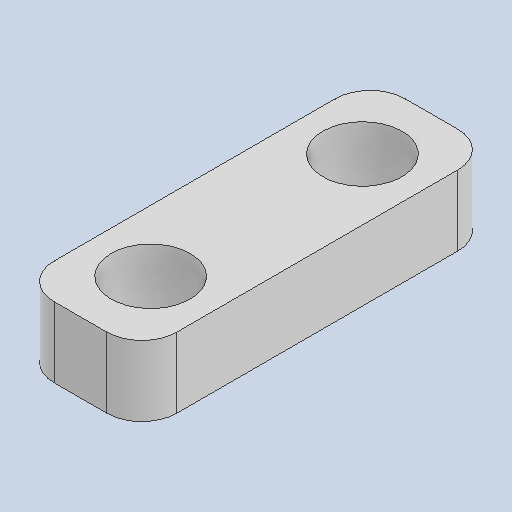
# Autodesk Inventor part: Aparter
Saved by Autodesk Inventor 2025 (Build 290162000, 162)
## iProperties
Created: 2025-08-11
Part Number: Aparter
Material: Generic
Document SubType Name: Modeling
Designer: Pravoslav
Density: 1 g/cm^3
Appearance: Default
Author: Pravoslav
Autodesk Inventor part; units mm, degrees
ref_plane "YZ Plane" through (0, 0, 0) normal (1, 0, 0) x (0, 1, 0)
ref_plane "XZ Plane" through (0, 0, 0) normal (0, 1, 0) x (-1, 0, 0)
ref_plane "XY Plane" through (0, 0, 0) normal (0, 0, 1) x (1, 0, 0)
sketch "Sketch1" plane through (0, 0, 0) normal (0, 1, 0) x (-1, 0, 0)
  circle A0 centre (-0.5725, 7.3819) radius 2.25
  circle A1 centre (-0.5725, -4.6791) radius 2.25
  line L0 (2.9275, 11.3819) -> (-4.0725, 11.3819)
  line L1 (-4.0725, 11.3819) -> (-4.0725, -8.6181)
  line L2 (-4.0725, -8.6181) -> (2.9275, -8.6181)
  line L3 (2.9275, -8.6181) -> (2.9275, 11.3819)
  point P0 (0, 0)
  dimension "d0" = 4.5
  dimension "d1" = 4.5
  dimension "d2" = 12.061
  dimension "d3" = 7
  dimension "d4" = 3.5
  dimension "d5" = 20
  dimension "d6" = 4
  constraints: 8 end point, 2 centre point, 2 parallel, 1 horizontal, 1 perpendicular
  measures "d0" diameter of A0
  measures "d1" diameter of A1
  measures "d2" distance of A1.centre A0.centre
  measures "d3" distance between parallel lines of L1 L3
  measures "d4" distance from line of L3 A0.centre
  measures "d5" distance between parallel lines of L2 L0
  measures "d6" distance from line of A0.centre L0
extrude "Extrusion1" add sketch "Sketch1" along normal blind 4
fillet "Fillet1" radius 2 4 edges at (-2.9275, 2, 11.3819) (4.0725, 2, 11.3819) (4.0725, 2, -8.6181) (-2.9275, 2, -8.6181)
body "Solid1"
